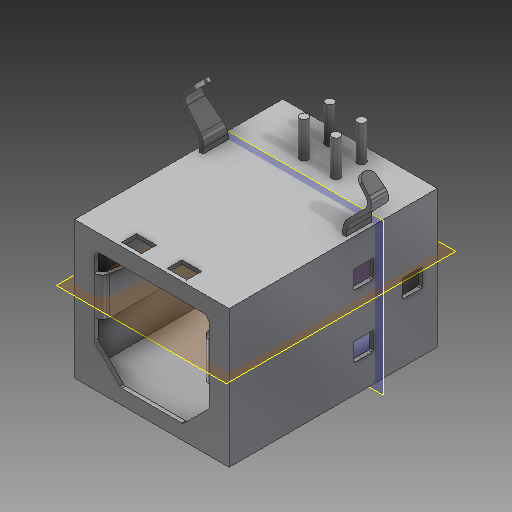
# Autodesk Inventor part: USB Series B Receptacle Metal Shel
Saved by Autodesk Inventor 2017 SP1 (Build 210196100, 196)
## iProperties
Created: 2012-05-07
Material: Copper
Document SubType Name: Modeling
Designer: sdarley
Density: 8.94 g/cm^3
Project: USB Series B Receptacle
Description: USB Series B Receptacle Metal Shel
Appearance: Metal
Author: sdarley
Title: USB Series B Receptacle Metal Shel
Revision Number: 1
Autodesk Inventor part; units mm, degrees
ref_plane "YZ Plane" through (0, 0, 0) normal (1, 0, 0) x (0, 1, 0)
ref_plane "XY Plane" through (0, 0, 0) normal (0, 0, 1) x (1, 0, 0)
sketch "Sketch1" plane through (0, 0, 0) normal (0, 0, 1) x (1, 0, 0)
  line L0 (-6.05, -5.375) -> (6.05, -5.375)
  line L1 (6.05, -5.375) -> (6.05, 5.375)
  line L2 (6.05, 5.375) -> (-6.05, 5.375)
  line L3 (-6.05, 5.375) -> (-6.05, -5.375)
  line L4 (-6.05, -5.375) -> (6.05, 5.375) construction
  line L5 (6.05, -5.375) -> (-6.05, 5.375) construction
  line L6 (4.5, 4.075) -> (-4.5, 4.075)
  line L7 (-4.5, 4.075) -> (-4.5, -2.175)
  line L8 (-4.5, -2.175) -> (-2.45, -4.225)
  line L9 (-2.45, -4.225) -> (2.45, -4.225)
  line L10 (2.45, -4.225) -> (4.5, -2.175)
  line L11 (4.5, -2.175) -> (4.5, 4.075)
  point P0 (0, 0)
  point P1 (0, -4.225)
  point P2 (0, -5.375)
  point P3 (0, 4.075)
  dimension "d0" = 12.1
  dimension "d1" = 10.75
  dimension "d2" = 8.3
  dimension "d3" = 9
  dimension "d4" = 1.3
  dimension "d5" = 4.9
  dimension "d6" = 6.25
  constraints: 24 end point, 5 midpoint, 4 parallel, 3 perpendicular, 2 vertical alignment, 1 horizontal, 1 horizontal alignment
  measures "d0" distance of L2.end L1.end
  measures "d1" distance of L1.end L0.end
  measures "d2" distance between parallel lines of L6 L9
  measures "d3" distance between parallel lines of L7 L11
  measures "d4" distance between parallel lines of L2 L6
  measures "d5" distance of L8.end L9.end
  measures "d6" distance of L6.end L7.end
extrude "Extrusion1" add sketch "Sketch1" along normal blind 0.3
sketch "Sketch2" plane through (0, 0, 0) normal (0, 0, -1) x (-1, 0, 0)
  line L0 (6.05, -5.375) -> (-6.05, -5.375) projected
  line L1 (6.05, 5.375) -> (6.05, -5.375) projected
  line L2 (-6.05, 5.375) -> (6.05, 5.375) projected
  line L3 (-6.05, -5.375) -> (-6.05, 5.375) projected
  line L4 (5.75, 5.075) -> (5.75, -5.075)
  line L5 (5.75, -5.075) -> (-5.75, -5.075)
  line L6 (-5.75, -5.075) -> (-5.75, 5.075)
  line L7 (-5.75, 5.075) -> (5.75, 5.075)
  point P0 (0, 0)
  dimension "d9" = 0.3
  constraints: 8 end point, 3 other
  measures "d9" distance between parallel lines of L2 L7
extrude "Extrusion2" add sketch "Sketch2" along normal blind 16
sketch "Sketch3" plane through (0, 0, -16) normal (0, 0, -1) x (-1, 0, 0)
  line L0 (5.75, -5.075) -> (-5.75, -5.075) projected
  line L1 (-5.75, -5.075) -> (-5.75, 5.075) projected
  line L2 (-5.75, 5.075) -> (5.75, 5.075) projected
  line L3 (5.75, 5.075) -> (5.75, -5.075) projected
  point P0 (0, 0)
extrude "Extrusion3" add sketch "Sketch3" against normal blind 0.3
fillet "Fillet1" radius 0.5 2 edges at (4.5, 4.075, 0.15) (-4.5, 4.075, 0.15)
fillet "Fillet2" radius 0.2 4 edges at (4.5, -2.175, 0.15) (2.45, -4.225, 0.15) (-2.45, -4.225, 0.15) (-4.5, -2.175, 0.15)
sketch "Sketch4" plane through (-6.05, -5.375, 0.3) normal (-1, 0, 0) x (0, 0, 1)
  line L0 (0, 0) -> (-16.3, 0) projected
  line L1 (-16.3, 10.75) -> (0, 10.75) projected
  line L2 (-16.3, 0) -> (-16.3, 10.75) projected
  line L3 (-9.85, 2.2) -> (-11.2, 2.2)
  line L4 (-11.3, 2.3) -> (-11.3, 3.55)
  line L5 (-11.2, 3.65) -> (-9.85, 3.65)
  line L6 (-9.75, 3.55) -> (-9.75, 2.3)
  line L7 (-9.85, 7.1) -> (-11.2, 7.1)
  line L8 (-11.3, 7.2) -> (-11.3, 8.45)
  line L9 (-11.2, 8.55) -> (-9.85, 8.55)
  line L10 (-9.75, 8.45) -> (-9.75, 7.2)
  line L11 (-13.65, 4.6) -> (-15, 4.6)
  line L12 (-15.1, 4.7) -> (-15.1, 5.95)
  line L13 (-15, 6.05) -> (-13.65, 6.05)
  line L14 (-13.55, 5.95) -> (-13.55, 4.7)
  arc A0 (-13.55, 5.95) -> (-13.65, 6.05) centre (-13.65, 5.95) ccw
  arc A1 (-15, 6.05) -> (-15.1, 5.95) centre (-15, 5.95) ccw
  arc A2 (-15.1, 4.7) -> (-15, 4.6) centre (-15, 4.7) ccw
  arc A3 (-13.65, 4.6) -> (-13.55, 4.7) centre (-13.65, 4.7) ccw
  arc A4 (-11.2, 3.65) -> (-11.3, 3.55) centre (-11.2, 3.55) ccw
  arc A5 (-11.3, 2.3) -> (-11.2, 2.2) centre (-11.2, 2.3) ccw
  arc A6 (-9.85, 2.2) -> (-9.75, 2.3) centre (-9.85, 2.3) ccw
  arc A7 (-9.75, 3.55) -> (-9.85, 3.65) centre (-9.85, 3.55) ccw
  arc A8 (-11.3, 7.2) -> (-11.2, 7.1) centre (-11.2, 7.2) ccw
  arc A9 (-9.85, 7.1) -> (-9.75, 7.2) centre (-9.85, 7.2) ccw
  arc A10 (-9.75, 8.45) -> (-9.85, 8.55) centre (-9.85, 8.45) ccw
  arc A11 (-11.2, 8.55) -> (-11.3, 8.45) centre (-11.2, 8.45) ccw
  point P0 (-9.75, 2.2)
  point P1 (-11.3, 3.65)
  point P2 (-11.3, 2.2)
  point P3 (-9.75, 3.65)
  point P4 (-9.75, 7.1)
  point P5 (-11.3, 8.55)
  point P6 (-11.3, 7.1)
  point P7 (-9.75, 8.55)
  point P8 (-13.55, 4.6)
  point P9 (-15.1, 6.05)
  point P10 (-15.1, 4.6)
  point P11 (-13.55, 6.05)
  dimension "d16" = 1.55
  dimension "d18" = 1.45
  dimension "d19" = 1.55
  dimension "d20" = 1.45
  dimension "d21" = 1.55
  dimension "d22" = 1.45
  dimension "d23" = 2.2
  dimension "d24" = 2.2
  dimension "d25" = 1.2
  dimension "d26" = 4.6
  dimension "d27" = 5
  dimension "d30" = 0.1
  constraints: 24 end point, 24 point on circle, 24 point on line, 24 tangent, 12 centre point, 11 equal radius, 6 parallel, 3 horizontal, 3 perpendicular, 1 vertical alignment
  measures "d16" distance of point (-9.75, 2.2) point (-11.3, 2.2)
  measures "d18" distance of point (-11.3, 2.2) point (-11.3, 3.65)
  measures "d19" distance of point (-9.75, 7.1) point (-11.3, 7.1)
  measures "d20" distance of point (-11.3, 7.1) point (-11.3, 8.55)
  measures "d21" distance of point (-13.55, 4.6) point (-15.1, 4.6)
  measures "d22" distance of point (-15.1, 4.6) point (-15.1, 6.05)
  measures "d23" distance between parallel lines of L0 L3
  measures "d24" distance between parallel lines of L1 L9
  measures "d25" distance between parallel lines of L2 L12
  measures "d26" distance between parallel lines of L0 L11
  measures "d27" distance between parallel lines of L2 L4
  measures "d30" radius of A0
extrude "Extrusion4" cut sketch "Sketch4" against normal through all
ref_plane "Work Plane1" through (0, 1, 0) normal (0, 1, 0) x (-1, 0, 0)
sketch "Sketch5" plane through (0, 1, 0) normal (0, 1, 0) x (-1, 0, 0)
  line L0 (6.05, 0.3) -> (-6.05, 0.3) projected
  line L1 (-4.5, 0.3) -> (-4.5, 0) projected
  line L2 (-5.75, 0) -> (5.75, 0) projected
  arc A0 (-3.8653, -0.284) -> (-4.5, 0.3) centre (-4.5, -0.3368) ccw
  arc A1 (-4.1643, -0.3089) -> (-4.5, 0) centre (-4.5, -0.3368) ccw
  line L3 (-4.1643, -0.3089) -> (-3.799, -4.7)
  line L4 (-3.799, -4.7) -> (-3.5, -4.6751)
  line L5 (-3.5, -4.6751) -> (-3.8653, -0.284)
  point P0 (0, 0)
  dimension "d32" = 5
  dimension "d33" = 1
  constraints: 6 end point, 4 point on circle, 4 tangent, 2 centre point, 1 concentric, 1 parallel, 1 perpendicular
  measures "d32" distance from line of L3.end L0
  measures "d33" distance from line of L4.end L1
extrude "Extrusion5" add sketch "Sketch5" along normal mid plane 3
sketch "Sketch6" plane through (3.8653, -0.5, -0.284) normal (-0.9965566, 0, 0.0829156) x (0.0829156, 0, 0.9965566)
  line L0 (0, 0) -> (0, 3) projected
  line L1 (-4.4063, 3) -> (0, 3) projected
  line L2 (-4.4063, 0) -> (-4.4063, 3) projected
  line L3 (0, 0) -> (-4.4063, 0) projected
  line L4 (0, 3) -> (-4.4063, 2.65)
  line L5 (-4.4063, 0.35) -> (0, 0)
  line L6 (-4.4063, 2.65) -> (-4.4063, 0.35)
  line L7 (0, 3) -> (0, 0)
  point P0 (-0.0374, 0.5)
  point P1 (-4.4063, 1.5)
  point P2 (0, 1.5)
  dimension "d36" = 2.3
  constraints: 8 end point, 2 midpoint, 2 point on line, 1 collinear, 1 horizontal alignment, 1 parallel
  measures "d36" distance of L4.end L5.start
extrude "Extrusion6" cut sketch "Sketch6" against normal up to next contours L3 L2 L5 | L4 L2 L1
mirror "Mirror1" about plane through (0, 0, 0) normal (1, 0, 0) of "Extrusion5", "Extrusion6"
sketch "Sketch7" plane through (-6.05, 5.375, 0.3) normal (0, 1, 0) x (1, 0, 0)
  line L0 (0, 16.3) -> (0, 0) projected
  line L1 (12.1, 0) -> (0, 0) projected
  line L2 (12.1, 16.3) -> (12.1, 0) projected
  line L3 (8.5, 0.3) -> (6.95, 0.3)
  line L4 (6.95, 0.3) -> (6.95, 1.45)
  line L5 (6.95, 1.45) -> (8.5, 1.45)
  line L6 (8.5, 1.45) -> (8.5, 0.3)
  line L7 (4.95, 0.3) -> (3.4, 0.3)
  line L8 (3.4, 0.3) -> (3.4, 1.45)
  line L9 (3.4, 1.45) -> (4.95, 1.45)
  line L10 (4.95, 1.45) -> (4.95, 0.3)
  dimension "d39" = 3.6
  dimension "d40" = 3.4
  dimension "d42" = 1.55
  dimension "d43" = 1.55
  dimension "d44" = 0.3
  dimension "d45" = 1.15
  constraints: 16 end point, 4 parallel, 2 horizontal, 2 horizontal alignment, 2 perpendicular
  measures "d39" distance between parallel lines of L2 L6
  measures "d40" distance between parallel lines of L0 L8
  measures "d42" distance of L3.start L3.end
  measures "d43" distance of L7.start L7.end
  measures "d44" distance between parallel lines of L1 L7
  measures "d45" distance of L5.end L3.start
extrude "Extrusion7" cut sketch "Sketch7" against normal up to next
ref_plane "Work Plane2" through (0, 0, -11.15) normal (0, 0, -1) x (-1, 0, 0)
sketch "Sketch8" plane through (0, 0, -11.15) normal (0, 0, -1) x (-1, 0, 0)
  line L0 (-6.05, -5.375) -> (6.05, -5.375) projected
  line L1 (6.05, -5.375) -> (6.05, 5.375) projected
  line L2 (6.05, 5.375) -> (-6.05, 5.375) projected
  line L3 (-6.05, 5.375) -> (-6.05, -5.375) projected
  line L4 (5.75, 5.375) -> (5.75, 5.768)
  line L5 (5.9843, 6.3337) -> (7.1907, 7.5401)
  line L6 (7.1907, 8.6714) -> (6.2671, 9.595)
  line L7 (6.2671, 9.595) -> (6.055, 9.3829)
  line L8 (6.055, 9.3829) -> (6.9786, 8.4593)
  line L9 (6.9786, 7.7522) -> (5.7722, 6.5458)
  line L10 (5.45, 5.768) -> (5.45, 5.375)
  line L11 (5.75, 5.375) -> (5.45, 5.375)
  arc A0 (6.9786, 7.7522) -> (6.9786, 8.4593) centre (6.625, 8.1058) ccw
  arc A1 (7.1907, 7.5401) -> (7.1907, 8.6714) centre (6.625, 8.1058) ccw
  line L12 (0, -5.375) -> (0, 5.375) construction
  arc A2 (5.9843, 6.3337) -> (5.75, 5.768) centre (6.55, 5.768) ccw
  arc A3 (5.7722, 6.5458) -> (5.45, 5.768) centre (6.55, 5.768) ccw
  point P0 (0, 0)
  dimension "d49" = 0.5
  dimension "d51" = 0.3
  dimension "d52" = 7.425
  dimension "d53" = 6.055
  dimension "d54" = 4.22
  dimension "d55" = 0.3
  dimension "d56" = 0.3
  dimension "d57" = 135
  dimension "d58" = 0.8
  dimension "d59" = 1.1
  constraints: 18 end point, 8 point on circle, 8 tangent, 5 parallel, 4 centre point, 2 midpoint, 2 perpendicular, 2 point on line, 1 concentric
  measures "d49" radius of A0
  measures "d51" distance between parallel lines of L8 L6
  measures "d53" distance from line of L12 L7.end
  measures "d54" distance from line of L6.end L2
  measures "d55" distance between parallel lines of L4 L10
  measures "d56" distance between parallel lines of L1 L4
  measures "d57" angle of L4 L5
  measures "d58" radius of A2
  measures "d59" radius of A3
extrude "Extrusion8" add sketch "Sketch8" against normal blind 2 contours L10 A3 L9 A0 L8 L7 L6 A1 L5 A2 L4 L2
sketch "Sketch9" plane through (-6.05, -5.375, 0.3) normal (-1, 0, 0) x (0, 0, 1)
  line L0 (-11.45, 14.97) -> (-9.45, 14.97) projected
  line L1 (-11.45, 10.75) -> (-11.45, 11.143) projected
  line L2 (-9.45, 11.143) -> (-9.45, 10.75) projected
  line L3 (-11.45, 10.75) -> (-10.9183, 14.97)
  line L4 (-9.45, 10.75) -> (-9.9183, 14.97)
  line L5 (-9.9183, 14.97) -> (-10.9183, 14.97)
  line L6 (-11.45, 10.75) -> (-11.45, 14.97)
  line L7 (-11.45, 14.97) -> (-9.45, 14.97)
  line L8 (-9.45, 10.75) -> (-9.45, 14.97)
  point P0 (-0.3, 5.375)
  point P1 (-10.45, 14.97)
  point P2 (-10.45, 14.97)
  dimension "d62" = 1
  constraints: 12 end point, 2 collinear, 2 midpoint, 2 perpendicular, 2 point on line, 1 coincident
  measures "d62" distance of L4.end L3.end
extrude "Extrusion9" cut sketch "Sketch9" along normal through all both and the other way through all
fillet "Fillet3" radius 0.55 2 edges at (-6.1611, 9.4889, -9.6066) (-6.1611, 9.4889, -10.6317)
mirror "Mirror2" about plane through (0, 0, 0) normal (1, 0, 0) of "Fillet3", "Extrusion9", "Extrusion8"
sketch "Sketch10" plane through (-6.05, 5.375, 0.3) normal (0, 1, 0) x (1, 0, 0)
  line L0 (0.6, 11.45) -> (0.6, 9.45) projected
  line L1 (0, 16.3) -> (12.1, 16.3) projected
  circle A0 centre (4.8, 15.16) radius 0.325
  circle A1 centre (7.3, 15.16) radius 0.325
  circle A2 centre (7.3, 13.16) radius 0.325
  circle A3 centre (4.8, 13.16) radius 0.325
  point P0 (6.05, 0.3)
  point P1 (0.6, 10.45)
  point P2 (6.05, 16.3)
  dimension "d66" = 2.71
  dimension "d67" = 0.65
  dimension "d68" = 4.71
  dimension "d69" = 2.5
  dimension "d70" = 1.25
  constraints: 4 centre point, 3 equal radius, 2 horizontal alignment, 2 midpoint, 2 vertical alignment
  measures "d66" vertical distance of A3.centre point (0.6, 10.45)
  measures "d67" diameter of A3
  measures "d68" vertical distance of A0.centre point (0.6, 10.45)
  measures "d69" distance of A1.centre A0.centre
  measures "d70" horizontal distance of point (6.05, 16.3) A0.centre
extrude "Extrusion10" add sketch "Sketch10" along normal blind 2.8
equation "\"d19\" = d16"
equation "\"d20\" = d18"
equation "\"d21\" = d16"
equation "\"d22\" = d18"
equation "\"d24\" = d23"
equation "\"d43\" = d42"
equation "\"d70\" = 0.5 * d69"
body "Solid1"
